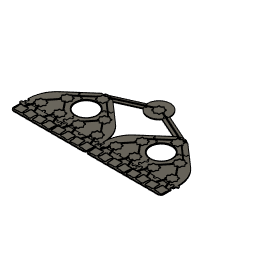
1 e 2- Base 8F e Raiz (Autodesk Fusion 360 design; units mm, degrees)
Autodesk Fusion 360 part; units mm, degrees
note: some values were not read from the file. Chosen so that the rebuilt part matches the saved one: which bodies a step acts on. Set by a fixed rule: which sketch regions a step uses.
(part 1 of 2)
sketch "Esboço1" plane through (0, 0, 0) normal (0, 0, 1) x (1, 0, 0)
  line L0 (-19, 19) -> (-19, -19)
  line L1 (-19, -19) -> (19, -19)
  line L2 (19, -19) -> (19, 19)
  line L3 (19, 19) -> (-19, -19) construction
  line L4 (-19, 19) -> (19, -19) construction
  line L5 (-20, -20) -> (20, -20)
  line L6 (20, -20) -> (20, 20)
  line L7 (20, 20) -> (-20, 20)
  line L8 (-20, 20) -> (-20, -20)
  line L9 (-119, -71) -> (-81, -109) construction
  line L10 (-120, -70) -> (-120, -110)
  line L11 (-120, -110) -> (-80, -110)
  line L12 (-80, -110) -> (-80, -70)
  line L13 (-80, -70) -> (-120, -70)
  line L14 (-81, -109) -> (-81, -71)
  line L15 (-81, -71) -> (-119, -109) construction
  line L16 (-119, -109) -> (-81, -109)
  line L17 (-81, -71) -> (-119, -71)
  line L18 (-119, -71) -> (-119, -109)
  line L19 (119, -71) -> (119, -109)
  line L20 (81, -71) -> (119, -71)
  line L21 (119, -71) -> (81, -109) construction
  line L22 (120, -70) -> (120, -110)
  line L23 (80, -110) -> (80, -70)
  line L24 (120, -110) -> (80, -110)
  line L25 (81, -109) -> (81, -71)
  line L26 (80, -70) -> (120, -70)
  line L27 (119, -109) -> (81, -109)
  line L28 (81, -71) -> (119, -109) construction
  line L29 (-169, -161) -> (-169, -199)
  line L30 (-169, -199) -> (-131, -199)
  line L31 (-131, -161) -> (-169, -199) construction
  line L32 (-130, -160) -> (-170, -160)
  line L33 (-130, -200) -> (-130, -160)
  line L34 (-131, -199) -> (-131, -161)
  line L35 (-169, -161) -> (-131, -199) construction
  line L36 (-170, -160) -> (-170, -200)
  line L37 (-170, -200) -> (-130, -200)
  line L38 (-131, -161) -> (-169, -161)
  line L39 (-100, -50) -> (-100, -260) construction
  line L40 (-69, -161) -> (-31, -199) construction
  line L41 (-69, -199) -> (-69, -161)
  line L42 (-70, -160) -> (-30, -160)
  line L43 (-69, -161) -> (-31, -161)
  line L44 (-70, -200) -> (-70, -160)
  line L45 (-30, -200) -> (-70, -200)
  line L46 (-31, -199) -> (-69, -199)
  line L47 (-30, -160) -> (-30, -200)
  line L48 (-31, -161) -> (-69, -199) construction
  line L49 (-31, -161) -> (-31, -199)
  line L50 (169, -199) -> (131, -199)
  line L51 (169, -161) -> (169, -199)
  line L52 (30, -200) -> (70, -200)
  line L53 (31, -161) -> (31, -199)
  line L54 (31, -161) -> (69, -199) construction
  line L55 (131, -199) -> (131, -161)
  line L56 (170, -200) -> (130, -200)
  line L57 (69, -161) -> (31, -161)
  line L58 (30, -160) -> (30, -200)
  line L59 (69, -161) -> (31, -199) construction
  line L60 (130, -200) -> (130, -160)
  line L61 (70, -160) -> (30, -160)
  line L62 (169, -161) -> (131, -199) construction
  line L63 (130, -160) -> (170, -160)
  line L64 (69, -199) -> (69, -161)
  line L65 (170, -160) -> (170, -200)
  line L66 (131, -161) -> (169, -199) construction
  line L67 (70, -200) -> (70, -160)
  line L68 (131, -161) -> (169, -161)
  line L69 (31, -199) -> (69, -199)
  line L70 (-195, -280) -> (-155, -280)
  line L71 (-195, -240) -> (-195, -280)
  line L72 (-156, -241) -> (-194, -279) construction
  line L73 (-155, -240) -> (-195, -240)
  line L74 (-194, -241) -> (-156, -279) construction
  line L75 (-155, -280) -> (-155, -240)
  line L76 (-150, -150.0869) -> (-150, -300) construction
  line L77 (-145, -280) -> (-145, -240)
  line L78 (-106, -241) -> (-144, -279) construction
  line L79 (-105, -280) -> (-145, -280)
  line L80 (-144, -241) -> (-106, -279) construction
  line L81 (-105, -240) -> (-105, -280)
  line L82 (-145, -240) -> (-105, -240)
  line L83 (-6, -241) -> (-44, -279) construction
  line L84 (-44, -241) -> (-6, -279) construction
  line L85 (-95, -240) -> (-95, -280)
  line L86 (-5, -280) -> (-45, -280)
  line L87 (-45, -240) -> (-5, -240)
  line L88 (-5, -240) -> (-5, -280)
  line L89 (-55, -280) -> (-55, -240)
  line L90 (-45, -280) -> (-45, -240)
  line L91 (-55, -240) -> (-95, -240)
  line L92 (-95, -280) -> (-55, -280)
  line L93 (-56, -241) -> (-94, -279) construction
  line L94 (-94, -241) -> (-56, -279) construction
  line L95 (-50, -150.0869) -> (-50, -300) construction
  line L96 (145, -240) -> (105, -240)
  line L97 (95, -280) -> (55, -280)
  line L98 (55, -240) -> (95, -240)
  line L99 (5, -280) -> (45, -280)
  line L100 (95, -240) -> (95, -280)
  line L101 (55, -280) -> (55, -240)
  line L102 (56, -241) -> (94, -279) construction
  line L103 (156, -241) -> (194, -279) construction
  line L104 (94, -241) -> (56, -279) construction
  line L105 (105, -280) -> (145, -280)
  line L106 (45, -280) -> (45, -240)
  line L107 (195, -240) -> (195, -280)
  line L108 (144, -241) -> (106, -279) construction
  line L109 (194, -241) -> (156, -279) construction
  line L110 (195, -280) -> (155, -280)
  line L111 (106, -241) -> (144, -279) construction
  line L112 (155, -280) -> (155, -240)
  line L113 (145, -280) -> (145, -240)
  line L114 (6, -241) -> (44, -279) construction
  line L115 (44, -241) -> (6, -279) construction
  line L116 (105, -240) -> (105, -280)
  line L117 (45, -240) -> (5, -240)
  line L118 (155, -240) -> (195, -240)
  line L119 (5, -240) -> (5, -280)
  line L120 (100, -70) -> (102.5, -70) construction
  line L121 (100, -70) -> (97.5, -70) construction
  line L122 (94.4216, -67.2941) -> (23.4089, -4.8754)
  line L123 (96.7606, -64.9552) -> (25.7479, -2.5364)
  line L124 (-94.4216, -67.2941) -> (-23.4089, -4.8754)
  line L125 (-50, -160) -> (-47.5, -160) construction
  line L126 (-50, -160) -> (-52.5, -160) construction
  line L127 (-100, -110) -> (-80, -110) construction
  line L128 (-52.5, -160) -> (-92.1676, -110.4518)
  line L129 (-47.5, -160) -> (-87.5293, -110)
  line L130 (-147.5, -160) -> (-107.8324, -110.4518)
  line L131 (-152.5, -160) -> (-112.4707, -110)
  line L132 (52.5, -160) -> (92.5293, -110)
  line L133 (47.5, -160) -> (87.5293, -110)
  line L134 (147.5, -160) -> (107.4707, -110)
  line L135 (152.5, -160) -> (112.4707, -110)
  line L136 (-150, -200) -> (-130, -200) construction
  line L137 (-150, -200) -> (-170, -200) construction
  line L138 (-125, -240) -> (-122.5, -240) construction
  line L139 (-125, -240) -> (-127.5, -240) construction
  line L140 (-122.5, -240) -> (-138, -200)
  line L141 (-127.8117, -239.1957) -> (-143, -200)
  line L142 (-172.1883, -239.1957) -> (-157, -200)
  line L143 (-177.5, -240) -> (-162, -200)
  line L144 (-22.5, -240) -> (-38, -200)
  line L145 (-27.8117, -239.1957) -> (-43, -200)
  line L146 (-72.1883, -239.1957) -> (-57, -200)
  line L147 (-77.5, -240) -> (-62, -200)
  line L148 (177.5, -240) -> (162, -200)
  line L149 (172.1883, -239.1957) -> (157, -200)
  line L150 (127.8117, -239.1957) -> (143, -200)
  line L151 (122.5, -240) -> (138, -200)
  line L152 (77.5, -240) -> (62, -200)
  line L153 (72.1883, -239.1957) -> (57, -200)
  line L154 (27.8117, -239.1957) -> (43, -200)
  line L155 (22.5, -240) -> (38, -200)
  line L156 (-185, -290) -> (185.016, -290)
  line L157 (148.7872, -80.1784) -> (32.9251, 21.1929)
  line L158 (-32.9239, 21.1916) -> (-148.7757, -80.1787)
  arc A0 (-148.7757, -80.1787) -> (-200, -193.0652) centre (-50, -193.0652) ccw
  arc A1 (200.016, -193.0688) -> (148.7872, -80.1784) centre (50.016, -193.0688) ccw
  arc A2 (-200, -275) -> (-185, -290) centre (-185, -275) ccw
  arc A3 (185.016, -290) -> (200.016, -275) centre (185.016, -275) ccw
  circle A4 centre (0, -87.6691) radius 60
  line L159 (-54.1918, -61.9154) -> (-56.9895, -59.4413)
  line L160 (-57.2096, -59.2467) -> (-56.9895, -59.4413)
  line L161 (-87.1239, -32.7932) -> (-90.8561, -29.4928)
  line L162 (87.1239, -32.7932) -> (90.8561, -29.4928)
  line L163 (54.1918, -61.9154) -> (56.9895, -59.4413)
  line L164 (57.2096, -59.2467) -> (56.9895, -59.4413)
  line L165 (0, -156.5102) -> (0, -147.6691)
  line L166 (0.0031, -202.4159) -> (0.0041, -221.188)
  line L167 (0.0049, -235.5875) -> (0.008, -290)
  line L168 (100, -260) -> (100, -117.7346) construction
  line L169 (200.016, -275) -> (200.016, -235.8808)
  line L170 (-200, -216.4079) -> (-194.408, -216.4079)
  line L171 (-200, -193.0652) -> (-200, -195.7356)
  line L172 (200.016, -220.8815) -> (200.016, -210.4308)
  line L173 (200.016, -196.0433) -> (200.016, -193.0688)
  line L174 (-20, -20) -> (20, -20)
  line L175 (20, -20) -> (20, 20)
  line L176 (19, -19) -> (19, 19)
  line L177 (-19, -19) -> (19, -19)
  line L178 (-19, 19) -> (-19, -19)
  line L179 (-20, 20) -> (-20, -20)
  line L180 (19, -106.6691) -> (-19, -106.6691)
  line L181 (-19, -106.6691) -> (-19, -68.6691)
  line L182 (-19, -68.6691) -> (19, -68.6691)
  line L183 (19, -68.6691) -> (19, -106.6691)
  line L184 (19, -106.6691) -> (-19, -68.6691) construction
  line L185 (-19, -106.6691) -> (19, -68.6691) construction
  line L186 (20, -107.6691) -> (-20, -107.6691)
  line L187 (-20, -107.6691) -> (-20, -67.6691)
  line L188 (-20, -67.6691) -> (20, -67.6691)
  line L189 (20, -67.6691) -> (20, -107.6691)
  line L190 (20, -107.6691) -> (-20, -67.6691) construction
  line L191 (-20, -107.6691) -> (20, -67.6691) construction
  line L192 (100, -70) -> (97.5, -70) construction
  line L193 (119, -71) -> (119, -109)
  line L194 (148.7872, -80.1784) -> (32.9251, 21.1929)
  circle A5 centre (0, -87.6691) radius 60
  line L195 (-20, -107.6691) -> (20, -67.6691) construction
  line L196 (80, -110) -> (80, -70)
  line L197 (20, -107.6691) -> (-20, -67.6691) construction
  line L198 (20, -67.6691) -> (20, -107.6691)
  line L199 (54.1918, -61.9154) -> (56.9895, -59.4413)
  line L200 (-19, -106.6691) -> (19, -68.6691) construction
  line L201 (19, -68.6691) -> (19, -106.6691)
  line L202 (120, -70) -> (120, -110)
  line L203 (20, -107.6691) -> (-20, -107.6691)
  line L204 (81, -109) -> (81, -71)
  line L205 (19, -106.6691) -> (-19, -68.6691) construction
  line L206 (147.5, -160) -> (107.4707, -110)
  line L207 (152.5, -160) -> (112.4707, -110)
  line L208 (47.5, -160) -> (87.5293, -110)
  line L209 (130, -160) -> (170, -160)
  line L210 (52.5, -160) -> (92.5293, -110)
  line L211 (131, -161) -> (169, -161)
  line L212 (119, -109) -> (81, -109)
  line L213 (100, -70) -> (102.5, -70) construction
  line L214 (-20, -20) -> (20, -20)
  line L215 (19, -106.6691) -> (-19, -106.6691)
  line L216 (96.7606, -64.9552) -> (25.7479, -2.5364)
  line L217 (57.2096, -59.2467) -> (56.9895, -59.4413)
  line L218 (100, -260) -> (100, -117.7346) construction
  line L219 (70, -160) -> (30, -160)
  line L220 (120, -110) -> (80, -110)
  line L221 (80, -70) -> (120, -70)
  line L222 (94.4216, -67.2941) -> (23.4089, -4.8754)
  line L223 (19, -19) -> (19, 19)
  line L224 (19, -19) -> (19, 19)
  line L225 (20, -20) -> (20, 20)
  line L226 (69, -161) -> (31, -161)
  line L227 (87.1239, -32.7932) -> (90.8561, -29.4928)
  line L228 (20, -20) -> (20, 20)
  line L229 (0, -156.5102) -> (0, -147.6691)
  line L230 (119, -71) -> (81, -109) construction
  line L231 (81, -71) -> (119, -109) construction
  line L232 (81, -71) -> (119, -71)
  line L233 (-20, -20) -> (20, -20)
  line L234 (-100, -50) -> (-100, -260) construction
  line L235 (45, -240) -> (5, -240)
  line L236 (0.0049, -235.5875) -> (0.008, -290)
  line L237 (-94, -241) -> (-56, -279) construction
  line L238 (55, -280) -> (55, -240)
  line L239 (-56, -241) -> (-94, -279) construction
  line L240 (5, -280) -> (45, -280)
  line L241 (-6, -241) -> (-44, -279) construction
  line L242 (-44, -241) -> (-6, -279) construction
  line L243 (0.0031, -202.4159) -> (0.0041, -221.188)
  line L244 (45, -280) -> (45, -240)
  line L245 (30, -200) -> (70, -200)
  line L246 (-50, -150.0869) -> (-50, -300) construction
  line L247 (56, -241) -> (94, -279) construction
  line L248 (77.5, -240) -> (62, -200)
  line L249 (94, -241) -> (56, -279) construction
  line L250 (5, -240) -> (5, -280)
  line L251 (22.5, -240) -> (38, -200)
  line L252 (72.1883, -239.1957) -> (57, -200)
  line L253 (27.8117, -239.1957) -> (43, -200)
  line L254 (169, -161) -> (169, -199)
  arc A6 (200.016, -193.0688) -> (148.7872, -80.1784) centre (50.016, -193.0688) ccw
  line L255 (30, -160) -> (30, -200)
  line L256 (31, -161) -> (31, -199)
  line L257 (95, -280) -> (55, -280)
  line L258 (170, -160) -> (170, -200)
  line L259 (55, -240) -> (95, -240)
  line L260 (130, -200) -> (130, -160)
  line L261 (69, -199) -> (69, -161)
  line L262 (131, -199) -> (131, -161)
  line L263 (70, -200) -> (70, -160)
  line L264 (-47.5, -160) -> (-87.5293, -110)
  line L265 (-120, -110) -> (-80, -110)
  line L266 (20, 20) -> (-20, 20)
  line L267 (-185, -290) -> (185.016, -290)
  line L268 (-19, -68.6691) -> (19, -68.6691)
  line L269 (-169, -161) -> (-131, -199) construction
  line L270 (-119, -109) -> (-81, -109)
  line L271 (-130, -160) -> (-170, -160)
  line L272 (-131, -161) -> (-169, -161)
  line L273 (-52.5, -160) -> (-92.1676, -110.4518)
  line L274 (-150, -200) -> (-170, -200) construction
  line L275 (6, -241) -> (44, -279) construction
  line L276 (44, -241) -> (6, -279) construction
  line L277 (-150, -150.0869) -> (-150, -300) construction
  line L278 (-70, -160) -> (-30, -160)
  line L279 (-150, -200) -> (-130, -200) construction
  line L280 (-147.5, -160) -> (-107.8324, -110.4518)
  line L281 (-152.5, -160) -> (-112.4707, -110)
  line L282 (-69, -161) -> (-31, -161)
  line L283 (-19, -19) -> (19, -19)
  arc A7 (185.016, -290) -> (200.016, -275) centre (185.016, -275) ccw
  line L284 (172.1883, -239.1957) -> (157, -200)
  line L285 (127.8117, -239.1957) -> (143, -200)
  line L286 (200.016, -220.8815) -> (200.016, -210.4308)
  line L287 (195, -280) -> (155, -280)
  line L288 (155, -240) -> (195, -240)
  line L289 (-100, -110) -> (-80, -110) construction
  line L290 (145, -280) -> (145, -240)
  line L291 (195, -240) -> (195, -280)
  line L292 (169, -199) -> (131, -199)
  line L293 (170, -200) -> (130, -200)
  line L294 (131, -161) -> (169, -199) construction
  line L295 (169, -161) -> (131, -199) construction
  line L296 (105, -240) -> (105, -280)
  line L297 (-119, -71) -> (-81, -109) construction
  line L298 (-81, -71) -> (-119, -109) construction
  line L299 (200.016, -196.0433) -> (200.016, -193.0688)
  line L300 (-19, 19) -> (19, -19) construction
  line L301 (19, 19) -> (-19, -19) construction
  line L302 (122.5, -240) -> (138, -200)
  line L303 (177.5, -240) -> (162, -200)
  line L304 (200.016, -275) -> (200.016, -235.8808)
  line L305 (155, -280) -> (155, -240)
  line L306 (-125, -240) -> (-127.5, -240) construction
  line L307 (-96.7606, -64.9552) -> (-25.7479, -2.5364)
  line L308 (-94.4216, -67.2941) -> (-23.4089, -4.8754)
  line L309 (-19, 19) -> (-19, -19)
  line L310 (-80, -70) -> (-120, -70)
  line L311 (-156, -241) -> (-194, -279) construction
  line L312 (-81, -71) -> (-119, -71)
  line L313 (-19, -19) -> (19, -19)
  line L314 (-20, 20) -> (-20, -20)
  line L315 (-87.1239, -32.7932) -> (-90.8561, -29.4928)
  line L316 (-194, -241) -> (-156, -279) construction
  line L317 (-20, -67.6691) -> (20, -67.6691)
  line L318 (-57.2096, -59.2467) -> (-56.9895, -59.4413)
  line L319 (-131, -161) -> (-169, -199) construction
  line L320 (-19, 19) -> (-19, -19)
  line L321 (-20, 20) -> (-20, -20)
  line L322 (-20, -107.6691) -> (-20, -67.6691)
  line L323 (-170, -160) -> (-170, -200)
  line L324 (-31, -199) -> (-69, -199)
  line L325 (-72.1883, -239.1957) -> (-57, -200)
  line L326 (-105, -280) -> (-145, -280)
  line L327 (-69, -199) -> (-69, -161)
  line L328 (-95, -240) -> (-95, -280)
  line L329 (-120, -70) -> (-120, -110)
  line L330 (-145, -240) -> (-105, -240)
  line L331 (-32.9239, 21.1916) -> (-148.7757, -80.1787)
  line L332 (-106, -241) -> (-144, -279) construction
  line L333 (-172.1883, -239.1957) -> (-157, -200)
  line L334 (-70, -200) -> (-70, -160)
  line L335 (-131, -199) -> (-131, -161)
  line L336 (-125, -240) -> (-122.5, -240) construction
  line L337 (-127.8117, -239.1957) -> (-143, -200)
  line L338 (-122.5, -240) -> (-138, -200)
  line L339 (-200, -216.4079) -> (-194.408, -216.4079)
  line L340 (-30, -200) -> (-70, -200)
  arc A8 (-148.7757, -80.1787) -> (-200, -193.0652) centre (-50, -193.0652) ccw
  line L341 (-55, -240) -> (-95, -240)
  line L342 (-130, -200) -> (-130, -160)
  line L343 (-31, -161) -> (-31, -199)
  line L344 (-30, -160) -> (-30, -200)
  line L345 (-54.1918, -61.9154) -> (-56.9895, -59.4413)
  line L346 (-119, -71) -> (-119, -109)
  line L347 (-144, -241) -> (-106, -279) construction
  line L348 (-27.8117, -239.1957) -> (-43, -200)
  line L349 (-169, -161) -> (-169, -199)
  line L350 (-177.5, -240) -> (-162, -200)
  line L351 (-19, -106.6691) -> (-19, -68.6691)
  line L352 (-81, -109) -> (-81, -71)
  line L353 (-77.5, -240) -> (-62, -200)
  line L354 (-22.5, -240) -> (-38, -200)
  line L355 (-80, -110) -> (-80, -70)
  line L356 (-200, -193.0652) -> (-200, -195.7356)
  line L357 (-170, -200) -> (-130, -200)
  line L358 (-145, -280) -> (-145, -240)
  line L359 (-105, -240) -> (-105, -280)
  line L360 (-5, -280) -> (-45, -280)
  line L361 (-195, -280) -> (-155, -280)
  line L362 (-195, -240) -> (-195, -280)
  line L363 (-55, -280) -> (-55, -240)
  line L364 (-169, -199) -> (-131, -199)
  line L365 (-155, -240) -> (-195, -240)
  line L366 (-95, -280) -> (-55, -280)
  line L367 (-45, -240) -> (-5, -240)
  line L368 (-45, -280) -> (-45, -240)
  line L369 (-5, -240) -> (-5, -280)
  line L370 (-155, -280) -> (-155, -240)
  arc A9 (-200, -275) -> (-185, -290) centre (-185, -275) ccw
  line L371 (95, -240) -> (95, -280)
  line L372 (194, -241) -> (156, -279) construction
  line L373 (31, -161) -> (69, -199) construction
  line L374 (106, -241) -> (144, -279) construction
  line L375 (144, -241) -> (106, -279) construction
  line L376 (-50, -160) -> (-52.5, -160) construction
  line L377 (105, -280) -> (145, -280)
  line L378 (145, -240) -> (105, -240)
  line L379 (69, -161) -> (31, -199) construction
  line L380 (156, -241) -> (194, -279) construction
  line L381 (-69, -161) -> (-31, -199) construction
  line L382 (-50, -160) -> (-47.5, -160) construction
  line L383 (-31, -161) -> (-69, -199) construction
  line L384 (31, -199) -> (69, -199)
  arc A10 (372.8384, 25.4826) -> (385.928, 31.4896) centre (379.4426, 28.3566) ccw
  line L385 (399.9966, 33.5625) -> (259.8581, 96.0843)
  arc A11 (372.8182, 25.5291) -> (367.0753, 21.1925) centre (399.9992, -16.4375) ccw
  line L386 (180, 80.2083) -> (180, 120.2083)
  line L387 (181, 119.2083) -> (181, 81.2083)
  line L388 (181, 81.2083) -> (219, 81.2083)
  line L389 (180, 120.2083) -> (220, 120.2083)
  line L390 (180, 80.2083) -> (220, 120.2083) construction
  line L391 (386.0569, 25.5059) -> (220, 100.2083)
  line L392 (385.906, 31.5352) -> (385.928, 31.4896)
  line L393 (181, 119.2083) -> (219, 81.2083) construction
  line L394 (200, 148.191) -> (200, 60.1906) construction
  arc A12 (258.8541, 88.5378) -> (141.1459, 88.5378) centre (200, 100.2083) ccw
  line L395 (219, 119.2083) -> (181, 119.2083)
  line L396 (220, 80.2083) -> (180, 80.2083)
  line L397 (220, 80.2083) -> (180, 120.2083) construction
  line L398 (383.0453, 22.1199) -> (220, 95.4694)
  line L399 (372.8182, 25.5291) -> (372.8384, 25.4826)
  arc A13 (145.9326, 74.1944) -> (254.0674, 74.1944) centre (200, 100.2083) ccw
  line L400 (259.8581, 96.0843) -> (259.8565, 96.085)
  line L401 (219, 119.2083) -> (181, 81.2083) construction
  arc A14 (399.9966, 33.5625) -> (385.906, 31.5352) centre (399.9992, -16.4375) ccw
  line L402 (361.6893, 16.4801) -> (367.0753, 21.1925)
  line L403 (361.6893, 16.4801) -> (249.6215, 66.4784)
  line L404 (0.0034, 33.5625) -> (140.1419, 96.0843)
  line L405 (6.2551, 22.0292) -> (180, 100.2083)
  line L406 (38.3107, 16.4801) -> (150.3785, 66.4784)
  line L407 (12.2772, 20) -> (180, 95.4694)
  line L408 (219, 81.2083) -> (219, 119.2083)
  line L409 (220, 120.2083) -> (220, 80.2083)
  arc A15 (32.9251, 21.1929) -> (27.182, 25.5295) centre (0.0013, -16.4373) ccw
  arc A16 (32.9251, 21.1929) -> (27.182, 25.5295) centre (0.0013, -16.4373) ccw
  line L410 (-27.1616, 25.4826) -> (-27.182, 25.5295)
  line L411 (-14.072, 31.4896) -> (-14.0942, 31.5355)
  arc A17 (14.0942, 31.5355) -> (-14.0939, 31.5349) centre (0.0013, -16.4373) ccw
  arc A18 (-27.1814, 25.5282) -> (-32.9239, 21.1916) centre (0.0013, -16.4373) ccw
  arc A19 (14.0942, 31.5355) -> (-14.0939, 31.5349) centre (0.0013, -16.4373) ccw
  arc A20 (-27.1814, 25.5282) -> (-32.9239, 21.1916) centre (0.0013, -16.4373) ccw
  circle A21 centre (0, -87.6691) radius 57
  line L412 (-54.1918, -61.9154) -> (-51.848, -63.9881)
  line L413 (20, -67.6691) -> (20, -107.6691)
  line L414 (-20, -107.6691) -> (-20, -67.6691)
  line L415 (-20, -107.6691) -> (20, -67.6691) construction
  line L416 (19, -106.6691) -> (-19, -68.6691) construction
  line L417 (-20, -107.6691) -> (20, -67.6691) construction
  line L418 (-20, -107.6691) -> (-20, -67.6691)
  line L419 (-19, -106.6691) -> (-19, -68.6691)
  line L420 (19, -106.6691) -> (-19, -68.6691) construction
  line L421 (-19, -106.6691) -> (19, -68.6691) construction
  line L422 (-19, -106.6691) -> (-19, -68.6691)
  line L423 (20, -67.6691) -> (20, -107.6691)
  line L424 (20, -107.6691) -> (-20, -67.6691) construction
  line L425 (-19, -106.6691) -> (19, -68.6691) construction
  line L426 (20, -107.6691) -> (-20, -67.6691) construction
  line L427 (19, -68.6691) -> (19, -106.6691)
  line L428 (-19, -68.6691) -> (19, -68.6691)
  line L429 (19, -68.6691) -> (19, -106.6691)
  line L430 (19, -106.6691) -> (-19, -106.6691)
  line L431 (19, -106.6691) -> (-19, -106.6691)
  line L432 (-19, -68.6691) -> (19, -68.6691)
  line L433 (20, -107.6691) -> (-20, -107.6691)
  line L434 (20, -107.6691) -> (-20, -107.6691)
  line L435 (-20, -67.6691) -> (20, -67.6691)
  line L436 (-20, -67.6691) -> (20, -67.6691)
  line L437 (20, -67.6691) -> (20, -107.6691)
  line L438 (-20, -107.6691) -> (-20, -67.6691)
  line L439 (-20, -107.6691) -> (20, -67.6691) construction
  line L440 (19, -106.6691) -> (-19, -68.6691) construction
  line L441 (-20, -107.6691) -> (20, -67.6691) construction
  line L442 (-20, -107.6691) -> (-20, -67.6691)
  line L443 (-19, -106.6691) -> (-19, -68.6691)
  line L444 (19, -106.6691) -> (-19, -68.6691) construction
  line L445 (-19, -106.6691) -> (19, -68.6691) construction
  line L446 (-19, -106.6691) -> (-19, -68.6691)
  line L447 (20, -67.6691) -> (20, -107.6691)
  line L448 (20, -107.6691) -> (-20, -67.6691) construction
  line L449 (-19, -106.6691) -> (19, -68.6691) construction
  line L450 (20, -107.6691) -> (-20, -67.6691) construction
  line L451 (19, -68.6691) -> (19, -106.6691)
  line L452 (-19, -68.6691) -> (19, -68.6691)
  line L453 (19, -68.6691) -> (19, -106.6691)
  line L454 (19, -106.6691) -> (-19, -106.6691)
  line L455 (19, -106.6691) -> (-19, -106.6691)
  line L456 (-19, -68.6691) -> (19, -68.6691)
  line L457 (20, -107.6691) -> (-20, -107.6691)
  line L458 (20, -107.6691) -> (-20, -107.6691)
  line L459 (-20, -67.6691) -> (20, -67.6691)
  line L460 (-20, -67.6691) -> (20, -67.6691)
  line L461 (20, -67.6691) -> (20, -107.6691)
  line L462 (-20, -107.6691) -> (-20, -67.6691)
  line L463 (-20, -107.6691) -> (20, -67.6691) construction
  line L464 (19, -106.6691) -> (-19, -68.6691) construction
  line L465 (-20, -107.6691) -> (20, -67.6691) construction
  line L466 (-20, -107.6691) -> (-20, -67.6691)
  line L467 (-19, -106.6691) -> (-19, -68.6691)
  line L468 (19, -106.6691) -> (-19, -68.6691) construction
  line L469 (-19, -106.6691) -> (19, -68.6691) construction
  line L470 (-19, -106.6691) -> (-19, -68.6691)
  line L471 (20, -67.6691) -> (20, -107.6691)
  line L472 (20, -107.6691) -> (-20, -67.6691) construction
  line L473 (-19, -106.6691) -> (19, -68.6691) construction
  line L474 (20, -107.6691) -> (-20, -67.6691) construction
  line L475 (19, -68.6691) -> (19, -106.6691)
  line L476 (-19, -68.6691) -> (19, -68.6691)
  line L477 (19, -68.6691) -> (19, -106.6691)
  line L478 (19, -106.6691) -> (-19, -106.6691)
  line L479 (19, -106.6691) -> (-19, -106.6691)
  line L480 (-19, -68.6691) -> (19, -68.6691)
  line L481 (20, -107.6691) -> (-20, -107.6691)
  line L482 (20, -107.6691) -> (-20, -107.6691)
  line L483 (-20, -67.6691) -> (20, -67.6691)
  line L484 (-20, -67.6691) -> (20, -67.6691)
  line L485 (-28.2843, 0) -> (0, -28.2843)
  line L486 (0, -28.2843) -> (28.2843, 0)
  line L487 (0, -26.8701) -> (26.8701, 0)
  line L488 (-26.8701, 0) -> (0, -26.8701)
  line L489 (0, 26.8701) -> (-26.8701, 0)
  line L490 (0, 28.2843) -> (-28.2843, 0)
  line L491 (26.8701, 0) -> (0, 26.8701)
  line L492 (28.2843, 0) -> (0, 28.2843)
  line L493 (54.1918, -61.9154) -> (51.848, -63.9881)
  line L494 (0, -147.6691) -> (0, -144.6691)
  line L495 (-100, -61.7157) -> (-128.2843, -90)
  line L496 (-100, -63.1299) -> (-126.8701, -90)
  line L497 (-73.1299, -90) -> (-100, -63.1299)
  line L498 (-71.7157, -90) -> (-100, -61.7157)
  line L499 (-100, -118.2843) -> (-71.7157, -90)
  line L500 (-100, -116.8701) -> (-73.1299, -90)
  line L501 (-128.2843, -90) -> (-100, -118.2843)
  line L502 (-126.8701, -90) -> (-100, -116.8701)
  line L503 (126.8701, -90) -> (100, -116.8701)
  line L504 (128.2843, -90) -> (100, -118.2843)
  line L505 (100, -116.8701) -> (73.1299, -90)
  line L506 (100, -118.2843) -> (71.7157, -90)
  line L507 (73.1299, -90) -> (100, -63.1299)
  line L508 (71.7157, -90) -> (100, -61.7157)
  line L509 (100, -63.1299) -> (126.8701, -90)
  line L510 (100, -61.7157) -> (128.2843, -90)
  line L511 (-150, -151.7157) -> (-178.2843, -180)
  line L512 (-178.2843, -180) -> (-150, -208.2843)
  line L513 (-176.8701, -180) -> (-150, -206.8701)
  line L514 (-150, -153.1299) -> (-176.8701, -180)
  line L515 (-123.1299, -180) -> (-150, -153.1299)
  line L516 (-121.7157, -180) -> (-150, -151.7157)
  line L517 (-150, -206.8701) -> (-123.1299, -180)
  line L518 (-150, -208.2843) -> (-121.7157, -180)
  line L519 (-50, -208.2843) -> (-78.2843, -180)
  line L520 (-50, -206.8701) -> (-76.8701, -180)
  line L521 (-78.2843, -180) -> (-50, -151.7157)
  line L522 (-76.8701, -180) -> (-50, -153.1299)
  line L523 (-50, -153.1299) -> (-23.1299, -180)
  line L524 (-50, -151.7157) -> (-21.7157, -180)
  line L525 (-21.7157, -180) -> (-50, -208.2843)
  line L526 (-23.1299, -180) -> (-50, -206.8701)
  line L527 (150, -151.7157) -> (178.2843, -180)
  line L528 (150, -153.1299) -> (176.8701, -180)
  line L529 (176.8701, -180) -> (150, -206.8701)
  line L530 (178.2843, -180) -> (150, -208.2843)
  line L531 (150, -206.8701) -> (123.1299, -180)
  line L532 (150, -208.2843) -> (121.7157, -180)
  line L533 (123.1299, -180) -> (150, -153.1299)
  line L534 (121.7157, -180) -> (150, -151.7157)
  line L535 (50, -208.2843) -> (78.2843, -180)
  line L536 (50, -206.8701) -> (76.8701, -180)
  line L537 (78.2843, -180) -> (50, -151.7157)
  line L538 (76.8701, -180) -> (50, -153.1299)
  line L539 (50, -153.1299) -> (23.1299, -180)
  line L540 (50, -151.7157) -> (21.7157, -180)
  line L541 (23.1299, -180) -> (50, -206.8701)
  line L542 (21.7157, -180) -> (50, -208.2843)
  line L543 (-158.7768, -236.8309) -> (-198.1691, -243.7768)
  line L544 (-151.8309, -276.2232) -> (-158.7768, -236.8309)
  line L545 (-198.1691, -243.7768) -> (-191.2232, -283.1691)
  line L546 (-191.2232, -283.1691) -> (-151.8309, -276.2232)
  line L547 (-141.2232, -236.8309) -> (-101.8309, -243.7768)
  line L548 (-148.1691, -276.2232) -> (-141.2232, -236.8309)
  line L549 (-108.7768, -283.1691) -> (-148.1691, -276.2232)
  line L550 (-101.8309, -243.7768) -> (-108.7768, -283.1691)
  line L551 (-41.2232, -236.8309) -> (-1.8309, -243.7768)
  line L552 (-48.1691, -276.2232) -> (-41.2232, -236.8309)
  line L553 (-8.7768, -283.1691) -> (-48.1691, -276.2232)
  line L554 (-1.8309, -243.7768) -> (-8.7768, -283.1691)
  line L555 (-58.7768, -236.8309) -> (-98.1691, -243.7768)
  line L556 (-51.8309, -276.2232) -> (-58.7768, -236.8309)
  line L557 (-98.1691, -243.7768) -> (-91.2232, -283.1691)
  line L558 (-91.2232, -283.1691) -> (-51.8309, -276.2232)
  line L559 (-96.7606, -64.9552) -> (-25.7479, -2.5364)
  line L560 (158.7768, -236.8309) -> (198.1691, -243.7768)
  line L561 (151.8309, -276.2232) -> (158.7768, -236.8309)
  line L562 (198.1691, -243.7768) -> (191.2232, -283.1691)
  line L563 (191.2232, -283.1691) -> (151.8309, -276.2232)
  line L564 (148.1691, -276.2232) -> (141.2232, -236.8309)
  line L565 (108.7768, -283.1691) -> (148.1691, -276.2232)
  line L566 (141.2232, -236.8309) -> (101.8309, -243.7768)
  line L567 (101.8309, -243.7768) -> (108.7768, -283.1691)
  line L568 (98.1691, -243.7768) -> (91.2232, -283.1691)
  line L569 (58.7768, -236.8309) -> (98.1691, -243.7768)
  line L570 (51.8309, -276.2232) -> (58.7768, -236.8309)
  line L571 (91.2232, -283.1691) -> (51.8309, -276.2232)
  line L572 (48.1691, -276.2232) -> (41.2232, -236.8309)
  line L573 (41.2232, -236.8309) -> (1.8309, -243.7768)
  line L574 (1.8309, -243.7768) -> (8.7768, -283.1691)
  line L575 (8.7768, -283.1691) -> (48.1691, -276.2232)
  line L576 (200, 128.4926) -> (228.2843, 100.2083)
  line L577 (226.8701, 100.2083) -> (200, 127.0783)
  line L578 (200, 73.3382) -> (226.8701, 100.2083)
  line L579 (228.2843, 100.2083) -> (200, 71.924)
  line L580 (171.7157, 100.2083) -> (200, 128.4926)
  line L581 (200, 127.0783) -> (173.1299, 100.2083)
  line L582 (173.1299, 100.2083) -> (200, 73.3382)
  line L583 (200, 71.924) -> (171.7157, 100.2083)
  arc A22 (146.0817, 73.8869) -> (141.0804, 88.8732) centre (146.4027, 82.3217) ccw
  arc A23 (145.9326, 74.1944) -> (141.1459, 88.5378) centre (146.4027, 82.3217) ccw
  arc A24 (258.8541, 88.5378) -> (254.0674, 74.1944) centre (253.5973, 82.3217) ccw
  arc A25 (258.9196, 88.8732) -> (253.9183, 73.8869) centre (253.5973, 82.3217) ccw
  arc A26 (145.9326, 74.1944) -> (141.1459, 88.5378) centre (146.4027, 82.3217) ccw
  arc A27 (146.0817, 73.8869) -> (141.0804, 88.8732) centre (146.4027, 82.3217) ccw
  arc A28 (146.0817, 73.8869) -> (141.0804, 88.8732) centre (146.4027, 82.3217) ccw
  arc A29 (145.9326, 74.1944) -> (141.1459, 88.5378) centre (146.4027, 82.3217) ccw
  arc A30 (18.9788, 29.7972) -> (26.8457, 25.7452) centre (22, 26) ccw
  arc A31 (18.6642, 29.9268) -> (27.1337, 25.5608) centre (22, 26) ccw
  spline S0 degree 5 poles (27.182, 25.5295) (27.1149, 25.573) (27.0477, 25.6163) (26.9805, 25.6594) (26.9131, 25.7024) (26.8457, 25.7452) knots 0 0 0 0 0 0 0.027546 0.027546 0.027546 0.027546 0.027546 0.027546
  line L584 (26.8801, 25.7233) -> (26.8113, 25.767)
  spline S1 degree 5 poles (18.9788, 29.7972) (18.5556, 29.9731) (17.5951, 30.3605) (16.6246, 30.7245) (15.6436, 31.0625) (14.651, 31.372) (14.0942, 31.5355) knots 0.641141 0.641141 0.641141 0.641141 0.641141 0.641141 0.8 1 1 1 1 1 1
  line L585 (19.4705, 29.5928) -> (18.4872, 30.0015)
  arc A32 (-27.1337, 25.5608) -> (-18.6642, 29.9268) centre (-22, 26) ccw
  line L586 (-6.2551, 22.0292) -> (-16.9141, 26.8254)
  line L587 (-12.2772, 20) -> (-18.108, 22.6236)
  spline S2 degree 5 poles (-14.0939, 31.5349) (-14.6507, 31.3713) (-15.5779, 31.0822) (-16.4951, 30.7681) (-17.4029, 30.4312) (-18.302, 30.0736) (-18.6633, 29.9261) knots 0 0 0 0 0 0 0.2 0.335238 0.335238 0.335238 0.335238 0.335238 0.335238
  line L588 (-18.2031, 30.114) -> (-19.1236, 29.7381)
  spline S3 degree 5 poles (-27.1335, 25.5592) (-27.1431, 25.553) (-27.1527, 25.5468) (-27.1623, 25.5406) (-27.1718, 25.5344) (-27.1814, 25.5282) knots 0.996069 0.996069 0.996069 0.996069 0.996069 0.996069 1 1 1 1 1 1
  line L589 (-27.1286, 25.5623) -> (-27.1384, 25.556)
  arc A33 (-85.4059, -34.3124) -> (-78.6796, -40.2606) centre (-83.2625, -38.6657) ccw
  arc A34 (-85.6477, -34.0987) -> (-78.4379, -40.4743) centre (-83.2625, -38.6657) ccw
  arc A35 (-58.5733, -58.0408) -> (-65.7561, -51.689) centre (-60.9143, -53.4509) ccw
  arc A36 (-58.816, -57.8262) -> (-65.5134, -51.9036) centre (-60.9143, -53.4509) ccw
  spline S4 degree 5 poles (-58.816, -57.8262) (-58.4507, -58.1492) (-58.0854, -58.4723) (-57.7201, -58.7953) (-57.3548, -59.1183) (-56.9895, -59.4413) knots 0.93939 0.93939 0.93939 0.93939 0.93939 0.93939 1 1 1 1 1 1
  line L590 (-59.0023, -57.6615) -> (-58.6297, -57.9909)
  spline S5 degree 5 poles (-87.1239, -32.7932) (-86.7803, -33.097) (-86.4367, -33.4009) (-86.0931, -33.7047) (-85.7495, -34.0086) (-85.4059, -34.3124) knots 0 0 0 0 0 0 0.05701 0.05701 0.05701 0.05701 0.05701 0.05701
  line L591 (-85.5812, -34.1575) -> (-85.2307, -34.4674)
  spline S6 degree 5 poles (-78.6796, -40.2606) (-77.9577, -40.899) (-76.0304, -42.6033) (-73.3972, -44.9319) (-70.764, -47.2605) (-68.1307, -49.589) (-66.2194, -51.2793) (-65.5134, -51.9036) knots 0.280222 0.280222 0.280222 0.280222 0.280222 0.280222 0.4 0.6 0.717137 0.717137 0.717137 0.717137 0.717137 0.717137
  line L592 (-80.0226, -39.073) -> (-77.3367, -41.4482)
  line L593 (-66.8564, -50.716) -> (-64.1705, -53.0912)
  arc A37 (65.5134, -51.9036) -> (58.816, -57.8262) centre (60.9143, -53.4509) ccw
  arc A38 (65.7561, -51.689) -> (58.5733, -58.0408) centre (60.9143, -53.4509) ccw
  arc A39 (78.6796, -40.2606) -> (85.4059, -34.3124) centre (83.2625, -38.6657) ccw
  arc A40 (78.4379, -40.4743) -> (85.6477, -34.0987) centre (83.2625, -38.6657) ccw
  spline S7 degree 5 poles (56.9895, -59.4413) (57.3548, -59.1183) (57.7201, -58.7953) (58.0854, -58.4723) (58.4507, -58.1492) (58.816, -57.8262) knots 0 0 0 0 0 0 0.06061 0.06061 0.06061 0.06061 0.06061 0.06061
  line L594 (58.6297, -57.9909) -> (59.0023, -57.6615)
  line L595 (54.1918, -61.9154) -> (78.6796, -40.2606) construction
  line L596 (85.4059, -34.3124) -> (90.8561, -29.4928) construction
  spline S8 degree 5 poles (65.5134, -51.9036) (66.2194, -51.2793) (68.1307, -49.589) (70.764, -47.2605) (73.3972, -44.9319) (76.0304, -42.6033) (77.9577, -40.899) (78.6796, -40.2606) knots 0.282863 0.282863 0.282863 0.282863 0.282863 0.282863 0.4 0.6 0.719778 0.719778 0.719778 0.719778 0.719778 0.719778
  line L597 (64.1705, -53.0912) -> (66.8564, -50.716)
  line L598 (77.3367, -41.4482) -> (80.0226, -39.073)
  spline S9 degree 5 poles (85.4059, -34.3124) (85.7495, -34.0086) (86.0931, -33.7047) (86.4367, -33.4009) (86.7803, -33.097) (87.1239, -32.7932) knots 0.94299 0.94299 0.94299 0.94299 0.94299 0.94299 1 1 1 1 1 1
  line L599 (85.2307, -34.4674) -> (85.5812, -34.1575)
  arc A41 (-189.8239, -216.4079) -> (-179.2301, -216.4079) centre (-184.527, -220.3221) ccw
  arc A42 (-189.4459, -216.4079) -> (-179.6081, -216.4079) centre (-184.527, -220.3221) ccw
  line L600 (-194.408, -216.4079) -> (-189.4459, -216.4079)
  arc A43 (-20.7699, -216.4079) -> (-10.1761, -216.4079) centre (-15.473, -220.3221) ccw
  arc A44 (-20.3919, -216.4079) -> (-10.5541, -216.4079) centre (-15.473, -220.3221) ccw
  arc A45 (-95.0856, -216.4079) -> (-104.9684, -216.4079) centre (-100.027, -212.5221) ccw
  arc A46 (-94.7091, -216.4079) -> (-105.3448, -216.4079) centre (-100.027, -212.5221) ccw
  line L601 (-179.6081, -216.4079) -> (-104.9684, -216.4079)
  line L602 (-95.0856, -216.4079) -> (-20.3919, -216.4079)
  line L603 (-10.5541, -216.4079) -> (-5.592, -216.4079)
  line L604 (-5.592, -216.4079) -> (10.5541, -216.4079)
  line L605 (189.4459, -216.4079) -> (200.016, -216.4079)
  line L606 (20.3919, -216.4079) -> (95.0856, -216.4079)
  line L607 (104.9684, -216.4079) -> (179.6081, -216.4079)
  arc A47 (189.4459, -216.4079) -> (179.6081, -216.4079) centre (184.527, -212.4936) ccw
  arc A48 (189.8239, -216.4079) -> (179.2301, -216.4079) centre (184.527, -212.4936) ccw
  arc A49 (95.0856, -216.4079) -> (104.9684, -216.4079) centre (100.027, -220.2936) ccw
  arc A50 (94.7091, -216.4079) -> (105.3448, -216.4079) centre (100.027, -220.2936) ccw
  arc A51 (20.7699, -216.4079) -> (10.1761, -216.4079) centre (15.473, -212.4936) ccw
  arc A52 (20.3919, -216.4079) -> (10.5541, -216.4079) centre (15.473, -212.4936) ccw
  arc A53 (200.0127, -208.4126) -> (200.0127, -198.5747) centre (203.927, -203.4936) ccw
  spline S10 degree 5 poles (200.016, -196.0433) (200.016, -196.5491) (200.016, -197.0548) (200.016, -197.5606) (200.016, -198.0664) (200.016, -198.5721) knots 0 0 0 0 0 0 0.175767 0.175767 0.175767 0.175767 0.175767 0.175767
  line L608 (200.016, -198.3142) -> (200.016, -198.8301)
  spline S11 degree 5 poles (200.016, -208.4151) (200.016, -208.8183) (200.016, -209.2214) (200.016, -209.6245) (200.016, -210.0277) (200.016, -210.4308) knots 0.859904 0.859904 0.859904 0.859904 0.859904 0.859904 1 1 1 1 1 1
  line L609 (200.016, -208.2096) -> (200.016, -208.6207)
  arc A54 (200.0193, -224.0252) -> (200.0193, -234.619) centre (196.105, -229.3221) ccw
  spline S12 degree 5 poles (200.016, -220.8815) (200.016, -221.4814) (200.016, -222.1097) (200.016, -222.738) (200.016, -223.3662) (200.016, -223.9945) (200.016, -224.0228) knots 0 0 0 0 0 0 0.2 0.209432 0.209432 0.209432 0.209432 0.209432 0.209432
  line L610 (200.016, -223.7024) -> (200.016, -224.3432)
  spline S13 degree 5 poles (200.016, -234.6215) (200.016, -234.8733) (200.016, -235.1252) (200.016, -235.3771) (200.016, -235.6289) (200.016, -235.8808) knots 0.91604 0.91604 0.91604 0.91604 0.91604 0.91604 1 1 1 1 1 1
  line L611 (200.016, -234.493) -> (200.016, -234.7499)
  arc A55 (200.0127, -208.7906) -> (200.016, -208.793) centre (203.927, -203.4936) ccw
  arc A56 (200.016, -198.1943) -> (200.0127, -198.1967) centre (203.927, -203.4936) ccw
  arc A57 (-200, -208.7959) -> (-200, -198.1914) centre (-196.093, -203.4936) ccw
  arc A58 (-200.159, -224.2665) -> (-200.159, -234.3778) centre (-203.895, -229.3221) ccw
  line L612 (-200, -195.7356) -> (-200, -198.1914)
  line L613 (-200, -208.7959) -> (-200, -224.3879)
  line L614 (-200, -234.2563) -> (-200, -275)
  arc A59 (0, -234.2563) -> (0.1774, -224.2529) centre (3.895, -229.3221) ccw
  arc A60 (0.159, -234.3778) -> (0.159, -224.2665) centre (3.895, -229.3221) ccw
  line L615 (0.159, -224.2665) -> (0, -224.384)
  line L616 (0.159, -234.3778) -> (0, -234.2603)
  line L617 (0, -234.2603) -> (0, -300) construction
  line L618 (0, -234.2563) -> (0, -300) construction
  line L619 (0.0041, -221.188) -> (0.0043, -224.3808)
  line L620 (0.0049, -234.2639) -> (0.0049, -235.5875)
  arc A61 (0.0073, -192.5747) -> (0.0073, -202.4126) centre (-3.907, -197.4936) ccw
  arc A62 (0.0073, -192.1967) -> (0.0073, -202.7906) centre (-3.907, -197.4936) ccw
  arc A63 (0.0073, -192.5747) -> (0.0073, -202.4126) centre (-3.907, -197.4936) ccw
  arc A64 (0.0073, -192.1967) -> (0.0073, -202.7906) centre (-3.907, -197.4936) ccw
  arc A65 (-0.0073, -172.4126) -> (-0.0073, -162.5747) centre (3.907, -167.4936) ccw
  arc A66 (-0.0073, -172.7906) -> (-0.0073, -162.1967) centre (3.907, -167.4936) ccw
  line L621 (0, 50) -> (0, -162.569) construction
  line L622 (0, -156.5102) -> (0.0004, -162.5687)
  line L623 (0.0011, -172.4192) -> (0.0025, -192.5709)
  line L624 (0, -172.4183) -> (0, -192.569) construction
  line L625 (0, -202.4183) -> (0, -224.384) construction
  line L626 (19, 19) -> (7.8701, 19)
  line L627 (-7.8701, 19) -> (-19, 19)
  line L628 (19, 19) -> (7.8701, 19)
  line L629 (-7.8701, 19) -> (-19, 19)
  line L630 (19, 19) -> (7.8701, 19)
  line L631 (-7.8701, 19) -> (-19, 19)
  line L632 (19, 19) -> (7.8701, 19)
  line L633 (-7.8701, 19) -> (-19, 19)
  line L634 (20, 20) -> (6.8701, 20)
  line L635 (0, 20) -> (-20, 20)
  line L636 (20, 20) -> (6.8701, 20)
  line L637 (0, 20) -> (-20, 20)
  spline S14 degree 5 poles (-200.159, -224.2665) (-200.1526, -224.2712) (-200.1388, -224.2835) (-200.1156, -224.3101) (-200.0809, -224.3576) (-200.0386, -224.4144) (-200.0129, -224.4353) (-200.0023, -224.4241) (-200, -224.4024) (-200, -224.3879) knots 0 0 0 0 0 0 0.2 0.4 0.6 0.8 1 1 1 1 1 1
  spline S15 degree 5 poles (-200.159, -234.3778) (-200.1526, -234.373) (-200.1388, -234.3608) (-200.1156, -234.3341) (-200.0809, -234.2866) (-200.0386, -234.2298) (-200.0129, -234.209) (-200.0023, -234.2201) (-200, -234.2419) (-200, -234.2563) knots 0 0 0 0 0 0 0.2 0.4 0.6 0.8 1 1 1 1 1 1
  point P0 (-100, -90)
  point P1 (-100, -90)
  point P2 (100, -90)
  point P3 (100, -90)
  point P4 (-150, -180)
  point P5 (-150, -180)
  point P6 (-50, -180)
  point P7 (-50, -180)
  point P8 (50, -180)
  point P9 (150, -180)
  point P10 (150, -180)
  point P11 (50, -180)
  point P12 (-175, -260)
  point P13 (-175, -260)
  point P14 (-125, -260)
  point P15 (-125, -260)
  point P16 (-25, -260)
  point P17 (-75, -260)
  point P18 (-75, -260)
  point P19 (-25, -260)
  point P20 (175, -260)
  point P21 (25, -260)
  point P22 (125, -260)
  point P23 (175, -260)
  point P24 (75, -260)
  point P25 (100, -260)
  point P26 (25, -260)
  point P27 (75, -260)
  point P28 (125, -260)
  point P29 (-80, -90)
  point P30 (-90, -110)
  point P31 (-125, -240)
  point P32 (-175, -240)
  point P33 (-140, -200)
  point P34 (-160, -200)
  point P35 (0, -87.6691)
  point P36 (0, -87.6691)
  point P37 (0, -87.6691)
  point P38 (125, -260)
  point P39 (-90, -110)
  point P40 (25, -260)
  point P41 (75, -260)
  point P42 (175, -260)
  point P43 (75, -260)
  point P44 (175, -260)
  point P45 (125, -260)
  point P46 (25, -260)
  point P47 (100, -260)
  point P48 (-80, -90)
  point P49 (-125, -240)
  point P50 (-175, -240)
  point P51 (-140, -200)
  point P52 (-160, -200)
  point P53 (-100, -90)
  point P54 (-100, -90)
  point P55 (100, -90)
  point P56 (-150, -180)
  point P57 (-150, -180)
  point P58 (-50, -180)
  point P59 (100, -90)
  point P60 (50, -180)
  point P61 (-50, -180)
  point P62 (150, -180)
  point P63 (150, -180)
  point P64 (50, -180)
  point P65 (-175, -260)
  point P66 (-175, -260)
  point P67 (-125, -260)
  point P68 (-25, -260)
  point P69 (-75, -260)
  point P70 (-125, -260)
  point P71 (-25, -260)
  point P72 (-75, -260)
  point P73 (0, -87.6691)
  point P74 (200, 100.2083)
  point P75 (200, 100.2083)
  point P76 (0, -87.6691)
  point P77 (0, -87.6691)
  point P78 (0, -87.6691)
  point P79 (0, -87.6691)
  point P80 (0, -87.6691)
  point P81 (0, -87.6691)
  point P82 (0, -87.6691)
  point P83 (0, -87.6691)
  point P84 (0, -87.6691)
  point P85 (0, -87.6691)
  point P86 (0, -87.6691)
  point P87 (0, -87.6691)
  point P88 (0, -87.6691)
  point P89 (0, -87.6691)
  point P90 (0, -87.6691)
  point P91 (0, -87.6691)
  point P92 (0, -87.6691)
  point P93 (0, -87.6691)
  point P94 (0, -87.6691)
  point P95 (0, -87.6691)
  point P96 (0, -87.6691)
  dimension "d1" = 38
  dimension "d2" = 38
  dimension "d4" = 40
  dimension "d5" = 1
  dimension "d6" = 38
  dimension "d7" = 38
  dimension "d8" = 40
  dimension "d9" = 1
  dimension "d10" = 38
  dimension "d11" = 38
  dimension "d12" = 40
  dimension "d14" = 38
  dimension "d15" = 38
  dimension "d16" = 40
  dimension "d20" = 2.5
  dimension "d21" = 2.5
  dimension "d22" = 138.685
  dimension "d23" = 2.5
  dimension "d24" = 2.5
  dimension "d27" = 2.5
  dimension "d28" = 2.5
  dimension "d30" = 10
  dimension "d31" = 50
  dimension "d32" = 150
  dimension "d34" = 15
  dimension "d36" = 120
  dimension "d90" = 38
  dimension "d91" = 38
  dimension "d92" = 40
  dimension "d93" = 38
  dimension "d94" = 38
  dimension "d95" = 40
  dimension "d96" = 40
  dimension "d103" = 1
  dimension "d104" = 1
  dimension "d107" = 38
  dimension "d108" = 38
  dimension "d109" = 40
  dimension "d110" = 38
  dimension "d111" = 38
  dimension "d112" = 40
  dimension "d113" = 38
  dimension "d114" = 38
  dimension "d115" = 40
  dimension "d116" = 38
  dimension "d117" = 38
  dimension "d118" = 40
  dimension "d119" = 2.5
  dimension "d120" = 2.5
  dimension "d121" = 138.685
  dimension "d122" = 2.5
  dimension "d123" = 2.5
  dimension "d124" = 2.5
  dimension "d125" = 2.5
  dimension "d126" = 10
  dimension "d127" = 50
  dimension "d128" = 150
  dimension "d129" = 15
  dimension "d130" = 120
  dimension "d147" = 38
  dimension "d148" = 38
  dimension "d149" = 40
  dimension "d150" = 38
  dimension "d151" = 38
  dimension "d152" = 40
  dimension "d153" = 40
  dimension "d164" = 120
  dimension "d165" = 38
  dimension "d166" = 38
  dimension "d167" = 40
  dimension "d168" = 40
  dimension "d190" = -3
  dimension "d191" = 38
  dimension "d192" = 38
  dimension "d193" = 40
  dimension "d194" = 40
  dimension "d195" = 38
  dimension "d196" = 38
  dimension "d197" = 40
  dimension "d198" = 40
  dimension "d199" = 38
  dimension "d200" = 38
  dimension "d201" = 40
  dimension "d202" = 40
  dimension "d203" = 38
  dimension "d204" = 38
  dimension "d205" = 40
  dimension "d206" = 40
  dimension "d207" = 38
  dimension "d208" = 38
  dimension "d209" = 40
  dimension "d210" = 40
  dimension "d211" = 38
  dimension "d212" = 38
  dimension "d213" = 40
  dimension "d214" = 40
  dimension "d215" = 38
  dimension "d216" = 40
  dimension "d217" = 38
  dimension "d218" = 38
  dimension "d219" = 38
  dimension "d220" = 40
  dimension "d221" = 38
  dimension "d222" = 38
  dimension "d223" = 38
  dimension "d224" = 40
  dimension "d226" = 40
  dimension "d300" = 38
  dimension "d301" = 38
  dimension "d302" = 40
  dimension "d303" = 40
  dimension "d376" = 6.2862
  dimension "d377" = 6.5862
  constraint horizontal L630
  constraint perpendicular L0 L630
  constraint parallel L1 L630
  constraint parallel L0 L2
  constraint coincident L3 origin
  constraint coincident L4 origin
  constraint horizontal L17
  constraint perpendicular L17 L18
  constraint parallel L16 L17
  constraint parallel L14 L18
  constraint coincident P54 L15
  constraint coincident P54 L9
  constraint coincident P54 P53
  constraint horizontal L38
  constraint perpendicular L29 L38
  constraint parallel L30 L38
  constraint parallel L29 L34
  constraint coincident P57 L31
  constraint coincident P57 L35
  constraint coincident P57 P56
  constraint vertical L39
  constraint symmetric P57 L39 P61
  constraint symmetric L31.start L39 L40.start
  constraint symmetric L30.end L39 L41.start
  constraint symmetric L32.end L39 L42.end
  constraint symmetric L29.end L39 L40.end
  constraint symmetric L32.start L39 L42.start
  constraint symmetric L29.start L39 L43.end
  constraint symmetric L36.end L39 L45.start
  constraint symmetric L33.start L39 L44.start
  constraint coincident P66 L72
  constraint coincident P66 L74
  constraint coincident P66 P65
  constraint perpendicular L32 L76
  constraint symmetric P66 L76 P70
  constraint symmetric L72.start L76 L80.start
  constraint symmetric L74.end L76 L78.end
  constraint symmetric L71.start L76 L81.start
  constraint symmetric L72.end L76 L80.end
  constraint symmetric L73.start L76 L77.end
  constraint symmetric L74.start L76 L78.start
  constraint symmetric L70.start L76 L79.start
  constraint symmetric L70.end L76 L77.start
  constraint symmetric L39 P66 P71
  constraint symmetric L39 L72.start L84.start
  constraint symmetric L39 L74.end L83.end
  constraint symmetric L39 L71.start L87.end
  constraint symmetric L39 L72.end L84.end
  constraint symmetric L39 L73.start L87.start
  constraint symmetric L39 L74.start L83.start
  constraint symmetric L39 L70.start L86.start
  constraint symmetric L39 L70.end L86.end
  constraint symmetric L39 L76.start L95.start
  constraint symmetric L39 L76.end L95.end
  constraint symmetric L39 L78.end L94.end
  constraint symmetric L39 P70 P72
  constraint symmetric L39 L77.start L89.start
  constraint symmetric L39 L81.start L85.start
  constraint symmetric L39 L79.start L85.end
  constraint symmetric L39 L78.start L94.start
  constraint symmetric L39 L80.end L93.end
  constraint symmetric L39 L77.end L89.end
  constraint symmetric L39 L80.start L93.start
  constraint midpoint L26 L120.start
  constraint parallel L26 L120
  constraint parallel L26 L121
  constraint parallel L122 L123
  constraint midpoint L42 L125.start
  constraint perpendicular L95 L125
  constraint perpendicular L95 L126
  constraint midpoint L12 P48
  constraint midpoint L11 L127.start
  constraint midpoint L127 P39
  constraint coincident L127 L129.end
  constraint parallel L128 L129
  constraint symmetric L39 L125.end L131.start
  constraint symmetric L39 L126.end L130.start
  constraint symmetric L39 L129.end L131.end
  constraint midpoint L82 P49
  constraint midpoint L73 P50
  constraint midpoint L37 L136.start
  constraint midpoint L136 P51
  constraint midpoint L137 P52
  constraint coincident P49 P31
  constraint parallel L82 L138
  constraint parallel L82 L139
  constraint coincident L37 L140.end
  constraint coincident L136 L141.end
  constraint parallel L140 L141
  constraint symmetric L76 L138.end L143.start
  constraint symmetric L76 L140.end L143.end
  constraint symmetric L76 L141.end L142.end
  constraint symmetric L39 L138.end L147.start
  constraint symmetric L39 L140.end L147.end
  constraint symmetric L39 L141.end L146.end
  constraint symmetric L39 L142.end L145.end
  constraint symmetric L39 L143.start L144.start
  constraint symmetric L39 L143.end L144.end
  constraint perpendicular L156 L171
  constraint tangent L158 A16
  constraint tangent L157 A16
  constraint tangent L158 A0
  constraint tangent A0 L171
  constraint tangent L157 A1
  constraint tangent A1 L169
  constraint tangent A2 L171
  constraint tangent L156 A2
  constraint tangent L156 A3
  constraint tangent A3 L169
  constraint coincident L170.start L171
  constraint coincident A4 L163.start
  constraint midpoint L157 L162.end
  constraint midpoint L156 L167.end
  constraint coincident A4 L165.end
  constraint collinear L166 L167
  constraint coincident P47 P25
  constraint parallel L100 L168
  constraint coincident L172.start L169
  constraint collinear L169 L172
  constraint coincident L173.start L172
  constraint collinear L172 L173
  constraint horizontal L626
  constraint perpendicular L178 L626
  constraint parallel L177 L626
  constraint parallel L176 L178
  constraint horizontal L180
  constraint perpendicular L180 L181